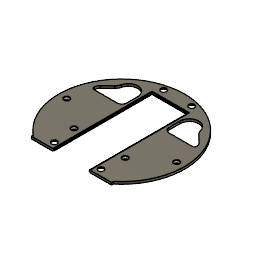
mid-2 (Autodesk Fusion 360 design; units mm, degrees)
Autodesk Fusion 360 part; units mm, degrees
sketch "Esboço5" plane through (0, 0, 0) normal (0, 1, 0) x (1, 0, 0)
  circle A0 centre (0, 0) radius 67.5
  dimension "d42" = 135
  constraint coincident A0.centre origin
  measures "d42" diameter of A0
extrude "Extrusão8" add sketch "Esboço5" along normal blind 2.5
sketch "Esboço6" plane through (0, 2.5, 0) normal (0, 1, 0) x (-1, 0, 0)
  circle A0 centre (0, 0) radius 67.5
  line L0 (0, 0) -> (0, -67.5) construction
  line L1 (0, 0) -> (-67.5, 0) construction
  line L2 (0, 0) -> (67.5, 0) construction
  line L3 (0, 0) -> (0, 67.5) construction
  line L4 (0, 67.5) -> (-20, 67.5)
  line L5 (0, 67.5) -> (20, 67.5)
  line L6 (20, 67.5) -> (20, -52.5)
  line L7 (20, -52.5) -> (-20, -52.5)
  line L8 (-20, -52.5) -> (-20, 67.5)
  line L9 (50, -17.9793) -> (25, -17.9793)
  line L10 (25, 0) -> (25, -17.9793)
  line L11 (55, -22.9793) -> (55, -27.9793)
  line L12 (55, -27.9793) -> (25, -27.9793)
  line L13 (25, -22.9793) -> (25, -27.9793)
  line L14 (40, -22.9793) -> (55, -22.9793)
  line L15 (25, -22.9793) -> (40, -22.9793)
  line L16 (-25, 27.0207) -> (-25, -17.9793)
  line L17 (55, 27.0207) -> (55, -18.0711)
  line L18 (55, -18.0711) -> (50, -17.9793)
  line L19 (25, 0) -> (25, 27.0207)
  line L20 (-55, 27.0207) -> (-55, -17.9793)
  line L21 (-25, -17.9793) -> (-55, -17.9793)
  circle A1 centre (32.7206, -39.8916) radius 10
  circle A2 centre (0, -60) radius 5.1214
  line L22 (-55, -22.9793) -> (-55, -27.9793)
  line L23 (-55, -27.9793) -> (-25, -27.9793)
  line L24 (-40, -22.9793) -> (-55, -22.9793)
  line L25 (-25, -22.9793) -> (-40, -22.9793)
  line L26 (-25, -22.9793) -> (-25, -27.9793)
  circle A3 centre (-32.7206, -39.8916) radius 10
  line L27 (25, 27.0207) -> (25, 42.0207)
  line L28 (25, 42.0207) -> (46.8502, 42.0207)
  line L29 (55, 27.0207) -> (46.8502, 42.0207)
  line L30 (-25, 27.0207) -> (-25, 42.0207)
  line L31 (-55, 27.0207) -> (-46.8502, 42.0207)
  line L32 (-25, 42.0207) -> (-46.8502, 42.0207)
  dimension "d47" = 120
  dimension "d48" = 40
  dimension "d63" = 20
  dimension "d65" = 15
  constraint coincident A0.centre L0.start
  constraint coincident A0 L0.end
  constraint vertical L0
  constraint coincident A0 L1.end
  constraint perpendicular L0 L1
  constraint coincident A0 L2.end
  constraint perpendicular L0 L2
  constraint coincident A0 L3.end
  constraint perpendicular L2 L3
  constraint perpendicular L3 L4
  constraint perpendicular L3 L5
  constraint perpendicular L5 L6
  constraint perpendicular L0 L7
  constraint coincident L2 L10.start
  constraint perpendicular L9 L10
  constraint perpendicular L9 L11
  constraint perpendicular L11 L12
  constraint perpendicular L12 L13
  constraint perpendicular L1 L16
  constraint symmetric L0 L14.start L24.start
  constraint symmetric L0 L11.end L22.end
  constraint symmetric L0 L12.end L23.end
  constraint symmetric L0 L11.start L22.start
  constraint symmetric L0 L13.start L25.start
  constraint symmetric L0 A1 A3
  constraint perpendicular L27 L28
  constraint symmetric L3 L19.end L16.start
  constraint symmetric L3 L17.start L20.start
  constraint symmetric L3 L27.end L30.end
  constraint symmetric L3 L28.end L31.end
  measures "d47" distance of L5.end L6.end
  measures "d48" distance of L6.end L7.end
  measures "d63" diameter of A1
  measures "d65" distance of L19.end L27.end
extrude "Extrusão9" cut sketch "Esboço6" against normal blind 10 contours A0 L6 L7 L8 | A1 | A2 | A3 picked at (0, -12.5)
extrude "Extrusão10" cut sketch "Esboço6" against normal blind 10 contours L11 L12 L13 L14 L15 | L22 L23 L24 L25 L26
extrude "Extrusão11" cut sketch "Esboço6" against normal blind 1 contours L9 L10 L17 L18 L19 L27 L28 L29 | L16 L20 L21 L30 L31 L32
sketch "Esboço7" plane through (0, 2.5, 0) normal (0, 1, 0) x (-1, 0, 0)
  line L0 (46.8502, 42.0207) -> (55, 27.0207)
  line L1 (55, 27.0207) -> (55, -18.0711)
  line L2 (55, -18.0711) -> (50, -17.9793)
  line L3 (50, -17.9793) -> (25, -17.9793)
  line L4 (25, -17.9793) -> (25, 42.0207)
  line L5 (25, 42.0207) -> (46.8502, 42.0207)
  line L6 (-46.8502, 42.0207) -> (-25, 42.0207)
  line L7 (-25, 42.0207) -> (-25, -17.9793)
  line L8 (-25, -17.9793) -> (-55, -17.9793)
  line L9 (-55, -17.9793) -> (-55, 27.0207)
  line L10 (-55, 27.0207) -> (-46.8502, 42.0207)
  line L11 (55, -27.9793) -> (25, -27.9793)
  line L12 (25, -27.9793) -> (25, -22.9793)
  line L13 (25, -22.9793) -> (55, -22.9793)
  line L14 (55, -22.9793) -> (55, -27.9793)
  line L15 (-55, -27.9793) -> (-55, -22.9793)
  line L16 (-55, -22.9793) -> (-25, -22.9793)
  line L17 (-25, -22.9793) -> (-25, -27.9793)
  line L18 (-25, -27.9793) -> (-55, -27.9793)
  line L19 (-20, -52.5) -> (-20, 64.469)
  arc A0 (-20, 64.469) -> (20, 64.469) centre (0, 0) ccw
  line L20 (20, 64.469) -> (20, -52.5)
  line L21 (20, -52.5) -> (-20, -52.5)
  circle A1 centre (32.7206, -39.8916) radius 10
  circle A2 centre (-32.7206, -39.8916) radius 10
  circle A3 centre (0, -60) radius 5.1214
  circle A4 centre (15, -60) radius 1.35
  circle A5 centre (15, -60) radius 3
  line L22 (0, -60) -> (0, 0) construction
  circle A6 centre (-15, -60) radius 1.35
  circle A7 centre (-15, -60) radius 3
  dimension "d72" = 15
  dimension "d74" = 2.7
  dimension "d78" = 6
  constraint concentric A4 A5
  constraint coincident A3.centre L22.start
  constraint coincident A0.centre L22.end
  constraint symmetric A4 L22 A6
  constraint symmetric A5 L22 A7
  measures "d72" distance of A3.centre A4.centre
  measures "d74" diameter of A4
  measures "d78" diameter of A5
extrude "Extrusão12" cut sketch "Esboço7" against normal blind 3 contours A4 | A5 | A6 | A7
sketch "Esboço8" plane through (0, 2.5, 0) normal (0, 1, 0) x (-1, 0, 0)
  circle A0 centre (15, -60) radius 3
  circle A1 centre (-15, -60) radius 3
  line L0 (46.8502, 42.0207) -> (55, 27.0207)
  line L1 (55, 27.0207) -> (55, -18.0711)
  line L2 (55, -18.0711) -> (50, -17.9793)
  line L3 (50, -17.9793) -> (25, -17.9793)
  line L4 (25, -17.9793) -> (25, 42.0207)
  line L5 (25, 42.0207) -> (46.8502, 42.0207)
  line L6 (-46.8502, 42.0207) -> (-25, 42.0207)
  line L7 (-25, 42.0207) -> (-25, -17.9793)
  line L8 (-25, -17.9793) -> (-55, -17.9793)
  line L9 (-55, -17.9793) -> (-55, 27.0207)
  line L10 (-55, 27.0207) -> (-46.8502, 42.0207)
  line L11 (55, -27.9793) -> (25, -27.9793)
  line L12 (25, -27.9793) -> (25, -22.9793)
  line L13 (25, -22.9793) -> (55, -22.9793)
  line L14 (55, -22.9793) -> (55, -27.9793)
  line L15 (-55, -27.9793) -> (-55, -22.9793)
  line L16 (-55, -22.9793) -> (-25, -22.9793)
  line L17 (-25, -22.9793) -> (-25, -27.9793)
  line L18 (-25, -27.9793) -> (-55, -27.9793)
  line L19 (-20, -52.5) -> (-20, 64.469)
  arc A2 (-20, 64.469) -> (20, 64.469) centre (0, 0) ccw
  line L20 (20, 64.469) -> (20, -52.5)
  line L21 (20, -52.5) -> (-20, -52.5)
  circle A3 centre (32.7206, -39.8916) radius 10
  circle A4 centre (-32.7206, -39.8916) radius 10
  circle A5 centre (0, -60) radius 5.1214
  line L22 (43.0128, 52.0207) -> (20, 52.0207)
  line L23 (-20, 52.0207) -> (-43.0128, 52.0207)
  constraint coincident A2 L22.start
  constraint coincident A2 L23.end
  constraint coincident L20 L22.end
  constraint coincident L19 L23.start
  constraint collinear L22 L23
extrude "Extrusão14" cut sketch "Esboço8" against normal blind 10 contours L19 A2 L23 | A2 L20 L22
sketch "Esboço10" plane through (0, 0, 0) normal (0, -1, 0) x (1, 0, 0)
  circle A0 centre (-32.7206, -39.8916) radius 10
  circle A1 centre (32.7206, -39.8916) radius 10
  circle A2 centre (0, -60) radius 5.1214
  line L0 (43.0128, 52.0207) -> (20, 52.0207)
  line L1 (20, 52.0207) -> (20, -52.5)
  line L2 (20, -52.5) -> (-20, -52.5)
  line L3 (-20, -52.5) -> (-20, 52.0207)
  line L4 (-20, 52.0207) -> (-43.0128, 52.0207)
  arc A3 (-43.0128, 52.0207) -> (43.0128, 52.0207) centre (0, 0) ccw
  line L5 (55, -22.9793) -> (55, -27.9793)
  line L6 (55, -27.9793) -> (25, -27.9793)
  line L7 (25, -27.9793) -> (25, -22.9793)
  line L8 (25, -22.9793) -> (55, -22.9793)
  line L9 (-25, -27.9793) -> (-55, -27.9793)
  line L10 (-55, -27.9793) -> (-55, -22.9793)
  line L11 (-55, -22.9793) -> (-25, -22.9793)
  line L12 (-25, -22.9793) -> (-25, -27.9793)
  circle A4 centre (15, -60) radius 3
  circle A5 centre (-15, -60) radius 3
  circle A6 centre (0, 0) radius 67.5
  line L13 (0, 0) -> (27.4835, 23.7231) construction
  line L14 (0, 0) -> (30.306, 0) construction
  circle A7 centre (27.4835, 23.7231) radius 1.5
  line L15 (0, 0) -> (0, 67.5) construction
  circle A8 centre (-27.4835, 23.7231) radius 1.5
  line L16 (0, 0) -> (67.5, 0) construction
  line L17 (67.5, 0) -> (58.987, 0) construction
  circle A9 centre (58.987, 0) radius 1.5
  circle A10 centre (-58.987, 0) radius 1.5
  dimension "d90" = 135
  dimension "d91" = 36.306
  dimension "d92" = 40.8
  dimension "d93" = 3
  dimension "d94" = 8.513
  dimension "d95" = 3
  constraint concentric A3 A6
  constraint horizontal L14
  constraint coincident A3.centre A6.centre
  constraint coincident L13.end A7.centre
  constraint coincident A6 L15.end
  constraint perpendicular L14 L15
  constraint symmetric A7 L15 A8
  constraint coincident A6 L16.end
  constraint coincident A3 L16.end
  constraint parallel L14 L16
  constraint parallel L16 L17
  constraint coincident L17.end A9.centre
  constraint symmetric L15 A9 A10
  measures "d90" diameter of A6
  measures "d91" distance of A3.centre L13.end
  measures "d92" angle of L13 L14
  measures "d93" diameter of A7
  measures "d94" distance of L16.end L17.end
  measures "d95" diameter of A9
sketch "Esboço11" plane through (0, 0, 0) normal (0, -1, 0) x (1, 0, 0)
  line L0 (0, 0) -> (-67.5, 0) construction
  line L1 (0, 0) -> (-20, 0) construction
  line L2 (-20, 0) -> (-25, 0) construction
  circle A0 centre (-25, 0) radius 2.5
  line L3 (0, 0) -> (0, 67.5) construction
  circle A1 centre (25, 0) radius 2.5
  dimension "d96" = 67.5
  dimension "d97" = 20
  dimension "d98" = 5
  dimension "d99" = 5
  dimension "d100" = 67.5
  constraint coincident L0.start L1.start
  constraint horizontal L0
  constraint parallel L0 L1
  constraint parallel L0 L2
  constraint coincident L2.end A0.centre
  constraint perpendicular L0 L3
  constraint symmetric A0 L3 A1
  measures "d96" distance of L0.start L0.end
  measures "d97" distance of L0.start L1.end
  measures "d98" distance of L1.end L2.end
  measures "d99" diameter of A0
  measures "d100" distance of L0.start L3.end
extrude "Extrusão15" cut sketch "Esboço11" against normal blind 3
extrude "Extrusão16" cut sketch "Esboço10" against normal blind 9 contours A7 | A8 | A9 | A10
extrude "Extrusão17" cut 1 faces at (29.3376, 2.5, 48.6874) along direction (0, -1, 0) blind 1
chamfer "Chanfro1" distance 1.5 angle 45 4 edges at (-60.3855, 1.5, 0.5424) (-28.882, 1.5, 23.1807) (26.085, 1.5, 23.1807) (57.5885, 1.5, 0.5424)
sketch "Esboço14" plane through (0, 1.5, 0) normal (0, 1, 0) x (-1, 0, 0)
  circle A0 centre (-27.4835, 23.7231) radius 3
  circle A1 centre (58.987, 0) radius 3
  circle A2 centre (-25, 0) radius 2.5
  circle A3 centre (0, -60) radius 5.1214
  circle A4 centre (-32.7206, -39.8916) radius 10
  circle A5 centre (32.7206, -39.8916) radius 10
  line L0 (-55, -27.9793) -> (-55, -22.9793)
  line L1 (-55, -22.9793) -> (-25, -22.9793)
  line L2 (-25, -22.9793) -> (-25, -27.9793)
  line L3 (-25, -27.9793) -> (-55, -27.9793)
  line L4 (55, -27.9793) -> (25, -27.9793)
  line L5 (25, -27.9793) -> (25, -22.9793)
  line L6 (25, -22.9793) -> (55, -22.9793)
  line L7 (55, -22.9793) -> (55, -27.9793)
  circle A6 centre (-15, -60) radius 3
  circle A7 centre (15, -60) radius 3
  line L8 (-20, 52.0207) -> (-43.0128, 52.0207)
  arc A8 (-43.0128, 52.0207) -> (43.0128, 52.0207) centre (0, 0) ccw
  line L9 (43.0128, 52.0207) -> (20, 52.0207)
  line L10 (20, 52.0207) -> (20, -52.5)
  line L11 (20, -52.5) -> (-20, -52.5)
  line L12 (-20, -52.5) -> (-20, 52.0207)
  circle A9 centre (25, 0) radius 2.5
  circle A10 centre (27.4835, 23.7231) radius 3
  circle A11 centre (-58.987, 0) radius 3
  circle A12 centre (25, 0) radius 2.5
  circle A13 centre (-25, 0) radius 2.5
  circle A14 centre (25, 47.2296) radius 3
  line L13 (0, 0) -> (0, 12.5091) construction
  circle A15 centre (-25, 47.2296) radius 3
  dimension "d110" = 6
  constraint concentric A9 A12
  constraint concentric A2 A13
  constraint coincident A8.centre L13.start
  constraint vertical L13
  constraint symmetric A14 L13 A15
  measures "d110" diameter of A14
extrude "Extrusão18" add sketch "Esboço14" against normal blind 1.5 contours A2 A13 | A9 A12
extrude "Extrusão19" cut sketch "Esboço14" against normal blind 2 contours A14 | A15
sketch "Esboço15" plane through (0, 0, 0) normal (0, -1, 0) x (1, 0, 0)
  circle A0 centre (-25, 47.2296) radius 3
  circle A1 centre (25, 47.2296) radius 3
  circle A2 centre (-58.987, 0) radius 1.5
  circle A3 centre (27.4835, 23.7231) radius 1.5
  circle A4 centre (-27.4835, 23.7231) radius 1.5
  circle A5 centre (58.987, 0) radius 1.5
  circle A6 centre (-32.7206, -39.8916) radius 10
  circle A7 centre (32.7206, -39.8916) radius 10
  circle A8 centre (0, -60) radius 5.1214
  line L0 (43.0128, 52.0207) -> (20, 52.0207)
  line L1 (20, 52.0207) -> (20, -52.5)
  line L2 (20, -52.5) -> (-20, -52.5)
  line L3 (-20, -52.5) -> (-20, 52.0207)
  line L4 (-20, 52.0207) -> (-43.0128, 52.0207)
  arc A9 (-43.0128, 52.0207) -> (43.0128, 52.0207) centre (0, 0) ccw
  line L5 (55, -22.9793) -> (55, -27.9793)
  line L6 (55, -27.9793) -> (25, -27.9793)
  line L7 (25, -27.9793) -> (25, -22.9793)
  line L8 (25, -22.9793) -> (55, -22.9793)
  line L9 (-25, -27.9793) -> (-55, -27.9793)
  line L10 (-55, -27.9793) -> (-55, -22.9793)
  line L11 (-55, -22.9793) -> (-25, -22.9793)
  line L12 (-25, -22.9793) -> (-25, -27.9793)
  circle A10 centre (15, -60) radius 3
  circle A11 centre (-15, -60) radius 3
  circle A12 centre (-25, 47.2296) radius 4.5
  circle A13 centre (25, 47.2296) radius 4.5
  circle A14 centre (-15, -60) radius 4.5
  circle A15 centre (15, -60) radius 4.5
  dimension "d115" = 9
  dimension "d116" = 9
  dimension "d117" = 9
  dimension "d118" = 9
  constraint concentric A0 A12
  constraint concentric A1 A13
  constraint concentric A11 A14
  constraint concentric A10 A15
  measures "d115" diameter of A12
  measures "d116" diameter of A13
  measures "d117" diameter of A14
  measures "d118" diameter of A15
extrude "Extrusão20" cut sketch "Esboço15" against normal blind 0.8 contours A12 | A13 | A14 | A15
sketch "Esboço16" plane through (0, 1.5, 0) normal (0, 1, 0) x (-1, 0, 0)
  circle A0 centre (25, 47.2296) radius 3
  circle A1 centre (-25, 47.2296) radius 3
  circle A2 centre (-27.4835, 23.7231) radius 3
  circle A3 centre (58.987, 0) radius 3
  circle A4 centre (0, -60) radius 5.1214
  circle A5 centre (-32.7206, -39.8916) radius 10
  circle A6 centre (32.7206, -39.8916) radius 10
  line L0 (-55, -27.9793) -> (-55, -22.9793)
  line L1 (-55, -22.9793) -> (-25, -22.9793)
  line L2 (-25, -22.9793) -> (-25, -27.9793)
  line L3 (-25, -27.9793) -> (-55, -27.9793)
  line L4 (55, -27.9793) -> (25, -27.9793)
  line L5 (25, -27.9793) -> (25, -22.9793)
  line L6 (25, -22.9793) -> (55, -22.9793)
  line L7 (55, -22.9793) -> (55, -27.9793)
  circle A7 centre (-15, -60) radius 3
  circle A8 centre (15, -60) radius 3
  line L8 (-20, 52.0207) -> (-43.0128, 52.0207)
  arc A9 (-43.0128, 52.0207) -> (43.0128, 52.0207) centre (0, 0) ccw
  line L9 (43.0128, 52.0207) -> (20, 52.0207)
  line L10 (20, 52.0207) -> (20, -52.5)
  line L11 (20, -52.5) -> (-20, -52.5)
  line L12 (-20, -52.5) -> (-20, 52.0207)
  circle A10 centre (27.4835, 23.7231) radius 3
  circle A11 centre (-58.987, 0) radius 3
  circle A12 centre (0, -60) radius 5.1214
  line L13 (32.7206, -39.8916) -> (22.7206, -39.8916)
  line L14 (22.7206, -39.8916) -> (22.7206, -22.9793)
  line L15 (25, -22.9793) -> (22.7206, -22.9793)
  line L16 (32.7206, -39.8916) -> (42.7206, -39.8916)
  line L17 (42.7206, -39.8916) -> (55, -27.9793)
  line L18 (0, 0) -> (0, -14.7997) construction
  line L19 (-22.7206, -39.8916) -> (-22.7206, -22.9793)
  line L20 (-25, -22.9793) -> (-22.7206, -22.9793)
  line L21 (-32.7206, -39.8916) -> (-42.7206, -39.8916)
  line L22 (-32.7206, -39.8916) -> (-22.7206, -39.8916)
  line L23 (-42.7206, -39.8916) -> (-55, -27.9793)
  constraint concentric A4 A12
  constraint coincident A6.centre L13.start
  constraint coincident A6 L13.end
  constraint perpendicular L5 L13
  constraint tangent A6 L14
  constraint coincident L5.end L6.start
  constraint perpendicular L14 L15
  constraint coincident L4.start L7.end
  constraint coincident A6 L16.end
  constraint parallel L13 L16
  constraint coincident A9.centre L18.start
  constraint vertical L18
  constraint symmetric A6.centre L18 A5.centre
  constraint symmetric L13.end L18 L19.start
  constraint symmetric L5.end L18 L1.end
  constraint symmetric L14.end L18 L19.end
  constraint symmetric L4.start L18 L0.start
  constraint symmetric L16.end L18 L21.end
extrude "Extrusão21" cut sketch "Esboço16" against normal blind 5 contours A5 L2 L3 L19 L20 L23 | A6 L4 L5 L14 L15 L17
extrude "Extrusão22" add sketch "Esboço16" against normal blind 1.5 contours A4 A12
extrude "Extrusão23" add 1 faces at (20, 1, -17.6598) along direction (-1, 0, 0) blind 1
extrude "Extrusão24" add 1 faces at (-20, 1, 17.1805) along direction (1, 0, 0) blind 1
extrude "Extrusão25" add 1 faces at (-6.3333, 1, -52.5) along direction (0, 0, 1) blind 1
extrude "Extrusão26" cut 4 faces at (-21.0279, 0.8, 46.857) (28.9721, 0.8, 46.857) (-11.0279, 0.8, -60.3726) (18.9721, 0.8, -60.3726) along direction (0, 1, 0) blind 0.2
fillet "Arredondamento1" radius 9.5 1 edges at (-42.7206, 0.75, -39.8916)
fillet "Arredondamento2" radius 9.5 1 edges at (42.7206, 0.75, -39.8916)
fillet "Arredondamento3" radius 6 1 edges at (-55, 0.75, -27.9793)
fillet "Arredondamento4" radius 6 1 edges at (55, 0.75, -27.9793)
fillet "Arredondamento5" radius 2 1 edges at (55, 0.75, -22.9793)
fillet "Arredondamento6" radius 2 1 edges at (-55, 0.75, -22.9793)
fillet "Arredondamento7" radius 5 1 edges at (-22.7206, 0.75, -22.9793)
fillet "Arredondamento8" radius 5 1 edges at (22.7206, 0.75, -22.9793)
sketch "Esboço17" plane through (0, 0, 0) normal (0, -1, 0) x (1, 0, 0)
  line L0 (43.0128, 52.0207) -> (19, 52.0207)
  line L1 (19, 52.0207) -> (19, -51.5)
  line L2 (19, -51.5) -> (-19, -51.5)
  line L3 (-19, -51.5) -> (-19, 52.0207)
  line L4 (-19, 52.0207) -> (-43.0128, 52.0207)
  arc A0 (-43.0128, 52.0207) -> (43.0128, 52.0207) centre (0, 0) ccw
  arc A1 (-42.4459, -42.2196) -> (-45.0701, -37.6124) centre (-51.6849, -44.4311) ccw
  line L5 (-45.0701, -37.6124) -> (-53.1778, -29.7471)
  arc A2 (-55, -25.4405) -> (-53.1778, -29.7471) centre (-49, -25.4405) ccw
  line L6 (-55, -25.4405) -> (-55, -24.9793)
  arc A3 (-53, -22.9793) -> (-55, -24.9793) centre (-53, -24.9793) ccw
  line L7 (-53, -22.9793) -> (-27.7206, -22.9793)
  arc A4 (-22.7206, -27.9793) -> (-27.7206, -22.9793) centre (-27.7206, -27.9793) ccw
  line L8 (-22.7206, -27.9793) -> (-22.7206, -39.8916)
  arc A5 (-42.4459, -42.2196) -> (-22.7206, -39.8916) centre (-32.7206, -39.8916) ccw
  circle A6 centre (58.987, 0) radius 1.5
  circle A7 centre (-27.4835, 23.7231) radius 1.5
  circle A8 centre (27.4835, 23.7231) radius 1.5
  circle A9 centre (-58.987, 0) radius 1.5
  circle A10 centre (15, -60) radius 4.5
  circle A11 centre (-25, 47.2296) radius 4.5
  circle A12 centre (-15, -60) radius 4.5
  circle A13 centre (25, 47.2296) radius 4.5
  arc A14 (45.0701, -37.6124) -> (42.4459, -42.2196) centre (51.6849, -44.4311) ccw
  arc A15 (22.7206, -39.8916) -> (42.4459, -42.2196) centre (32.7206, -39.8916) ccw
  line L9 (22.7206, -39.8916) -> (22.7206, -27.9793)
  arc A16 (27.7206, -22.9793) -> (22.7206, -27.9793) centre (27.7206, -27.9793) ccw
  line L10 (27.7206, -22.9793) -> (53, -22.9793)
  arc A17 (55, -24.9793) -> (53, -22.9793) centre (53, -24.9793) ccw
  line L11 (55, -24.9793) -> (55, -25.4405)
  arc A18 (53.1778, -29.7471) -> (55, -25.4405) centre (49, -25.4405) ccw
  line L12 (53.1778, -29.7471) -> (45.0701, -37.6124)
  line L13 (-19, 52.0207) -> (-20, 52.0207)
  line L14 (0, 0) -> (0, 16.459) construction
  line L15 (-20, 52.0207) -> (-20, -51.5)
  line L16 (-19, -52.5) -> (-20, -52.5)
  line L17 (-20, -51.5) -> (-20, -52.5)
  line L18 (-19, -52.5) -> (19, -52.5)
  line L19 (19, -52.5) -> (20, -52.5)
  line L20 (20, -52.5) -> (20, 52.0207)
  dimension "d149" = 1
  dimension "d150" = 1
  dimension "d151" = 1
  dimension "d152" = 1
  constraint coincident L3.end L4.start
  constraint perpendicular L3 L13
  constraint coincident A0.centre L14.start
  constraint vertical L14
  constraint perpendicular L13 L15
  constraint parallel L16 L18
  constraint coincident L0 L20.end
  constraint perpendicular L0 L20
  measures "d149" distance of L3.end L13.end
  measures "d150" distance of L2.end L16.start
  measures "d151" distance of L16.start L16.end
  measures "d152" distance of L18.end L19.end
extrude "Extrusão27" add sketch "Esboço17" along normal blind 0.5 contours L0 L4 A0 L15 L16 L17 L18 L19 L20
extrude "Extrusão28" add 4 faces at (35.3418, -0.3333, 52.0207) (27.3376, 1, 52.0207) (-35.3418, -0.3333, 52.0207) (-27.3376, 1, 52.0207) along direction (0, 0, 1) blind 2
extrude "Extrusão29" add 3 faces at (-35.0085, 1.5, 52.6874) (27.0043, 1.5, 52.6874) (37.2863, 1.5, -0.7269) along direction (0, 1, 0) blind 0.5
sketch "Esboço18" plane through (0, 0, 54.0207) normal (0, 0, 1) x (1, 0, 0)
  line L0 (-43.0128, 2) -> (-43.0128, -0.5)
  line L1 (-43.0128, -0.5) -> (-20, -0.5)
  line L2 (-20, -0.5) -> (-20, 0)
  line L3 (-20, 0) -> (-19, 0)
  line L4 (-19, 0) -> (-19, 2)
  line L5 (-19, 2) -> (-43.0128, 2)
  line L6 (-20, 0) -> (-20, 2)
  constraint coincident L2.end L3.start
  constraint coincident L5 L6.end
  constraint perpendicular L5 L6
sketch "Esboço19" plane through (0, 2, 0) normal (0, 1, 0) x (-1, 0, 0)
  arc A0 (-42.4459, -42.2196) -> (-45.0701, -37.6124) centre (-51.6849, -44.4311) ccw
  line L0 (-45.0701, -37.6124) -> (-53.1778, -29.7471)
  arc A1 (-55, -25.4405) -> (-53.1778, -29.7471) centre (-49, -25.4405) ccw
  line L1 (-55, -25.4405) -> (-55, -24.9793)
  arc A2 (-53, -22.9793) -> (-55, -24.9793) centre (-53, -24.9793) ccw
  line L2 (-53, -22.9793) -> (-27.7206, -22.9793)
  arc A3 (-22.7206, -27.9793) -> (-27.7206, -22.9793) centre (-27.7206, -27.9793) ccw
  line L3 (-22.7206, -27.9793) -> (-22.7206, -39.8916)
  arc A4 (-42.4459, -42.2196) -> (-22.7206, -39.8916) centre (-32.7206, -39.8916) ccw
  arc A5 (45.0701, -37.6124) -> (42.4459, -42.2196) centre (51.6849, -44.4311) ccw
  arc A6 (22.7206, -39.8916) -> (42.4459, -42.2196) centre (32.7206, -39.8916) ccw
  line L4 (22.7206, -39.8916) -> (22.7206, -27.9793)
  arc A7 (27.7206, -22.9793) -> (22.7206, -27.9793) centre (27.7206, -27.9793) ccw
  line L5 (27.7206, -22.9793) -> (53, -22.9793)
  arc A8 (55, -24.9793) -> (53, -22.9793) centre (53, -24.9793) ccw
  line L6 (55, -24.9793) -> (55, -25.4405)
  arc A9 (53.1778, -29.7471) -> (55, -25.4405) centre (49, -25.4405) ccw
  line L7 (53.1778, -29.7471) -> (45.0701, -37.6124)
  circle A10 centre (25, 47.2296) radius 3
  circle A11 centre (-25, 47.2296) radius 3
  circle A12 centre (-27.4835, 23.7231) radius 3
  circle A13 centre (58.987, 0) radius 3
  circle A14 centre (-15, -60) radius 3
  circle A15 centre (15, -60) radius 3
  arc A16 (-43.0128, 52.0207) -> (43.0128, 52.0207) centre (0, 0) ccw
  line L8 (43.0128, 52.0207) -> (43.0128, 54.0207)
  line L9 (43.0128, 54.0207) -> (19, 54.0207)
  line L10 (19, 54.0207) -> (19, -51.5)
  line L11 (19, -51.5) -> (-19, -51.5)
  line L12 (-19, -51.5) -> (-19, 54.0207)
  line L13 (-19, 54.0207) -> (-43.0128, 54.0207)
  line L14 (-43.0128, 54.0207) -> (-43.0128, 52.0207)
  circle A17 centre (27.4835, 23.7231) radius 3
  circle A18 centre (-58.987, 0) radius 3
  line L15 (0, 0) -> (0, 6.185) construction
  line L16 (19, 54.0207) -> (20, 54.0207)
  line L17 (20, 54.0207) -> (20, -52.5)
  line L18 (19, -52.5) -> (20, -52.5)
  line L19 (19, -52.5) -> (0, -52.5)
  line L20 (0, 0) -> (0, -52.5)
  line L21 (-19, -52.5) -> (0, -52.5)
  line L22 (-19, -52.5) -> (-20, -52.5)
  line L23 (-20, 54.0207) -> (-20, -52.5)
  dimension "d159" = 1
  dimension "d160" = 1
  constraint coincident A16.centre L15.start
  constraint vertical L15
  constraint coincident L9.end L10.start
  constraint perpendicular L10 L16
  constraint perpendicular L16 L17
  constraint perpendicular L17 L18
  constraint perpendicular L11 L20
  constraint symmetric L16.end L20 L23.start
  constraint symmetric L18.start L20 L21.start
  constraint symmetric L17.end L20 L22.end
  constraint symmetric L20 L19.end L21.end
  measures "d159" distance of L9.end L16.end
  measures "d160" distance of L10.end L18.start
extrude "Extrusão30" cut sketch "Esboço19" against normal blind 0.5 contours L11 L12 L13 L20 L21 L22 L23 | L9 L10 L11 L16 L17 L18 L19 L20
extrude "Extrusão13" [suppressed]
sketch "Esboço9" plane through (0, 0, 0) normal (0, -1, 0) x (1, 0, 0)
  circle A0 centre (-32.7206, -39.8916) radius 10
  circle A1 centre (32.7206, -39.8916) radius 10
  circle A2 centre (0, -60) radius 5.1214
  line L0 (-20, 52.0207) -> (-43.0128, 52.0207)
  arc A3 (-43.0128, 52.0207) -> (43.0128, 52.0207) centre (0, 0) ccw
  line L1 (43.0128, 52.0207) -> (20, 52.0207)
  line L2 (20, 52.0207) -> (20, -52.5)
  line L3 (20, -52.5) -> (-20, -52.5)
  line L4 (-20, -52.5) -> (-20, 52.0207)
  line L5 (55, -22.9793) -> (55, -27.9793)
  line L6 (55, -27.9793) -> (25, -27.9793)
  line L7 (25, -27.9793) -> (25, -22.9793)
  line L8 (25, -22.9793) -> (55, -22.9793)
  line L9 (-25, -27.9793) -> (-55, -27.9793)
  line L10 (-55, -27.9793) -> (-55, -22.9793)
  line L11 (-55, -22.9793) -> (-25, -22.9793)
  line L12 (-25, -22.9793) -> (-25, -27.9793)
  circle A4 centre (15, -60) radius 2.5
  circle A5 centre (-61.1758, 4.4748) radius 2.5
  circle A6 centre (-15, -60) radius 2.5
  circle A7 centre (61.1758, 4.4748) radius 2.5
  circle A8 centre (0, 0) radius 67.5
  line L13 (0, 0) -> (27.4835, 23.7231) construction
  line L14 (0, 0) -> (36.306, 0) construction
  circle A9 centre (27.4835, 23.7231) radius 2.5
  line L15 (0, 0) -> (0, 67.5) construction
  circle A10 centre (-27.4835, 23.7231) radius 2.5
  line L16 (-67.5, 0) -> (67.4997, 0.2003)
  dimension "d84" = 135
  dimension "d85" = 40.8
  dimension "d86" = 36.306
  dimension "d87" = 5
  constraint concentric A3 A8
  constraint horizontal L14
  constraint coincident A3.centre A8.centre
  constraint coincident L13.end A9.centre
  constraint coincident A8 L15.end
  constraint perpendicular L14 L15
  constraint symmetric A9 L15 A10
  constraint coincident A8 L16.start
  constraint coincident A3 L16.start
  constraint coincident A8 L16.end
  measures "d84" diameter of A8
  measures "d85" angle of L13 L14
  measures "d86" distance of A3.centre L13.end
  measures "d87" diameter of A9
equation "d96 = ( 135 / 2 ) * 1 mm"
equation "d100 = ( 135 / 2 ) * 1 mm"
